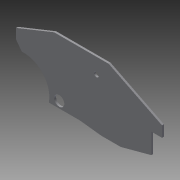
# Autodesk Inventor part: ShooterMountLeft_NERDS
Saved by Autodesk Inventor 2014 (Build 180170000, 170)
## iProperties
Created: 2016-01-30
Part Number: ShooterMountLeft_NERDS
Material: Generic
Document SubType Name: Modeling
Designer: bermudezr
Density: 1 g/cm^3
Appearance: Default
Author: bermudezr
Autodesk Inventor part; units mm, degrees
ref_plane "YZ Plane" through (0, 0, 0) normal (1, 0, 0) x (0, 1, 0)
ref_plane "XZ Plane" through (0, 0, 0) normal (0, 1, 0) x (-1, 0, 0)
ref_plane "XY Plane" through (0, 0, 0) normal (0, 0, 1) x (1, 0, 0)
sketch "Sketch1" plane through (0, 0, 0) normal (0, 0, 1) x (1, 0, 0)
  line L0 (-84.0821, 192.7052) -> (642.9929, 192.7052)
  line L1 (642.9929, 192.7052) -> (642.9929, -137.4948)
  line L2 (642.9929, -137.4948) -> (-84.0821, -137.4948)
  line L3 (-84.0821, -137.4948) -> (-84.0821, 192.7052)
  circle A0 centre (131.8179, -91.7748) radius 25.4
  circle A1 centre (318.0537, 116.5052) radius 12.7
  line L4 (642.9929, -137.4948) -> (592.1929, -137.4948)
  line L5 (592.1929, -137.4948) -> (592.1929, -73.9948)
  line L6 (592.1929, -73.9948) -> (642.9929, -73.9948)
  line L7 (642.9929, -73.9948) -> (642.9929, -137.4948)
  line L8 (642.9929, 192.7052) -> (592.6352, 192.7052)
  line L9 (642.9929, 2.2052) -> (642.9929, 192.7052)
  line L10 (-84.0821, 53.0052) -> (5.7204, 53.0052) construction
  line L11 (-84.0821, 65.7052) -> (68.3179, -137.4948)
  line L12 (595.3679, 192.7052) -> (595.3679, 2.2052)
  line L13 (595.3679, 2.2052) -> (642.9929, 2.2052)
  point P0 (0, 0)
  dimension "d0" = 727.075
  dimension "d2" = 50.8
  dimension "d3" = 25.4
  dimension "d4" = 215.9
  dimension "d5" = 279.4
  dimension "d14" = 152.4
  dimension "d15" = 203.2
  dimension "d16" = 330.2
  dimension "d17" = 63.5
  dimension "d19" = 50.8
  dimension "d20" = 139.7
  dimension "d21" = 45.72
  dimension "d22" = 254
  constraints: 28 end point, 5 parallel, 5 point on line, 4 horizontal, 3 perpendicular, 2 centre point
  measures "d0" distance of L1.end L2.end
  measures "d2" diameter of A0
  measures "d3" diameter of A1
  measures "d4" distance from line of L3 A0.centre
  measures "d5" distance of A1.centre A0.centre
  measures "d14" distance from line of L3 L11.end
  measures "d15" distance from line of L2 L11.start
  measures "d16" distance between parallel lines of L2 L0
  measures "d17" distance between parallel lines of L6 L2
  measures "d19" distance of L5.end L6.end
  measures "d20" distance between parallel lines of L13 L4
  measures "d21" distance from line of L2 A0.centre
  measures "d22" distance from line of L2 A1.centre
extrude "Extrusion1" add sketch "Sketch1" along normal blind 9.525 contours L0 L12 L13 L1 L6 L5 L2 L11 L3
sketch "Sketch3" plane through (0, 0, 9.525) normal (0, 0, 1) x (1, 0, 0)
  line L0 (595.3679, 2.2052) -> (595.3679, 192.7052) projected
  line L1 (595.3679, 192.7052) -> (-84.0821, 192.7052) projected
  line L2 (-84.0821, 192.7052) -> (-84.0821, 65.7052) projected
  line L3 (-84.0821, 116.5052) -> (106.4179, 192.7052)
  line L4 (595.3679, 2.2052) -> (684.2679, 2.2052)
  line L5 (684.2679, 2.2052) -> (684.2679, 40.3052)
  line L6 (684.2679, 40.3052) -> (595.3679, 40.3052)
  line L7 (595.3679, 40.3052) -> (595.3679, 2.2052)
  line L8 (684.2679, 40.3052) -> (379.4679, 192.7052)
  line L9 (595.3679, 40.3052) -> (595.3679, 84.7552)
  line L10 (595.3679, 84.7552) -> (595.3679, 192.7052)
  point P0 (0, 0)
  dimension "d32" = 190.5
  dimension "d33" = 76.2
  dimension "d38" = 88.9
  dimension "d39" = 38.1
  dimension "d40" = 215.9
  constraints: 16 end point, 5 point on line, 2 parallel, 1 collinear, 1 horizontal, 1 perpendicular
  measures "d32" distance from line of L2 L3.end
  measures "d33" distance from line of L1 L3.start
  measures "d38" distance of L6.end L5.end
  measures "d39" distance of L5.end L4.end
  measures "d40" distance of L0.end L8.end
extrude "Extrusion4" cut sketch "Sketch3" against normal blind 9.525 contours L8 L1 L0 | L0 L8 L6 | L3 L2 L1
sketch "Sketch4" plane through (0, 0, 9.525) normal (0, 0, 1) x (1, 0, 0)
  line L0 (595.3679, 2.2052) -> (595.3679, 84.7552) projected
  line L1 (595.3679, 84.7552) -> (379.4679, 192.7052) projected
  line L2 (595.3679, 84.7552) -> (684.2679, 40.3052)
  line L3 (684.2679, 40.3052) -> (595.3679, 40.3052)
  point P0 (0, 0)
  dimension "d43" = 88.9
  constraints: 4 end point, 1 collinear, 1 perpendicular, 1 point on line
  measures "d43" distance from line of L2.end L0
extrude "Extrusion5" add sketch "Sketch4" against normal blind 9.525
sketch "Sketch5" plane through (0, 0, 9.525) normal (0, 0, 1) x (1, 0, 0)
  line L0 (642.9929, 2.2052) -> (592.1929, 2.2052)
  line L1 (592.1929, 2.2052) -> (592.1929, -73.9948)
  line L2 (592.1929, -73.9948) -> (642.9929, -73.9948)
  line L3 (642.9929, -73.9948) -> (642.9929, 2.2052)
  point P0 (0, 0)
  constraints: 8 end point, 2 parallel, 1 horizontal, 1 perpendicular
extrude "Extrusion6" cut sketch "Sketch5" against normal blind 9.525
sketch "Sketch6" plane through (0, 0, 9.525) normal (0, 0, 1) x (1, 0, 0)
  line L0 (592.1929, -137.4948) -> (592.1929, 2.2052) projected
  line L1 (646.1679, 91.1052) -> (723.1394, 91.1052)
  line L2 (723.1394, 91.1052) -> (723.1394, -6.7385)
  line L3 (723.1394, -6.7385) -> (646.1679, -6.7385)
  line L4 (646.1679, -6.7385) -> (646.1679, 91.1052)
  line L5 (595.3679, 2.2052) -> (592.1929, 2.2052)
  line L6 (592.1929, 2.2052) -> (592.1929, 40.3052)
  line L7 (592.1929, 40.3052) -> (595.3679, 40.3052)
  line L8 (595.3679, 40.3052) -> (595.3679, 2.2052)
  point P0 (0, 0)
  dimension "d48" = 53.975
  constraints: 16 end point, 4 parallel, 2 horizontal, 2 perpendicular
  measures "d48" distance between parallel lines of L0 L4
extrude "Extrusion7" cut sketch "Sketch6" against normal blind 9.525
sketch "Sketch8" plane through (0, 0, 9.525) normal (0, 0, 1) x (1, 0, 0)
  line L0 (-84.0821, 65.7052) -> (68.3179, -137.4948) projected
  line L1 (68.3179, -137.4948) -> (592.1929, -137.4948) projected
  line L2 (592.1929, -137.4948) -> (592.1929, 40.3052) projected
  line L3 (592.1929, -96.6594) -> (439.7929, -137.4948)
  line L4 (341.7489, -137.4948) -> (170.3104, -117.1748)
  line L5 (170.3104, -117.1748) -> (53.0779, -117.1748)
  point P0 (0, 0)
  dimension "d51" = 152.4
  dimension "d52" = 165
  dimension "d53" = 98.044
  dimension "d54" = 20.32
  dimension "d60" = 173.24
  constraints: 6 end point, 4 point on line
  measures "d51" distance from line of L3.end L2
  measures "d52" angle of L1 L3
  measures "d53" distance of L3.end L4.start
  measures "d54" distance between parallel lines of L1 L5
  measures "d60" angle of L1 L4
extrude "Extrusion8" cut sketch "Sketch8" against normal blind 9.525
sketch "Sketch9" plane through (0, 0, 9.525) normal (0, 0, 1) x (1, 0, 0)
  line L0 (592.1929, -96.6594) -> (592.1929, 40.3052) projected
  line L1 (646.1679, 40.3052) -> (592.1929, 40.3052)
  line L2 (592.1929, 40.3052) -> (592.1929, 5.3802)
  line L3 (592.1929, 5.3802) -> (646.1679, 5.3802)
  line L4 (646.1679, 5.3802) -> (646.1679, 40.3052)
  point P0 (0, 0)
  dimension "d57" = 34.925
  constraints: 8 end point, 2 parallel, 1 horizontal, 1 perpendicular, 1 point on line
  measures "d57" distance of L2.end L1.end
extrude "Extrusion9" add sketch "Sketch9" against normal blind 9.525
sketch "Sketch10" plane through (0, 0, 9.525) normal (0, 0, 1) x (1, 0, 0)
  line L0 (-84.0821, 65.7052) -> (53.0779, -117.1748) projected
  line L1 (-84.0821, 116.5052) -> (-84.0821, 65.7052) projected
  line L2 (53.0779, -117.1748) -> (170.3104, -117.1748) projected
  arc A0 (81.0179, -117.1748) -> (-55.5071, 27.6052) centre (-44.6649, -98.9312) ccw
  point P0 (0, 0)
  point P1 (131.8179, -117.1748)
  dimension "d62" = 38.1
  dimension "d65" = 127
  dimension "d66" = 165.1
  constraints: 2 point on circle, 2 point on line, 1 centre point
  measures "d62" vertical distance of L0.start A0.end
  measures "d65" radius of A0
  measures "d66" distance from line of A0.start L1
extrude "Extrusion10" cut sketch "Sketch10" against normal blind 25.4
sketch "Sketch11" plane through (0, 0, 9.525) normal (0, 0, 1) x (1, 0, 0)
  arc A0 (81.0179, -117.1748) -> (-55.5071, 27.6052) centre (-44.6649, -98.9312) ccw projected
  line L0 (81.0179, -117.1748) -> (131.8179, -117.1748) projected
  line L1 (131.8179, -117.1748) -> (170.3104, -117.1748) projected
  line L2 (170.3104, -117.1748) -> (341.7489, -137.4948) projected
  line L3 (341.7489, -137.4948) -> (439.7929, -137.4948) projected
  line L4 (-84.0821, 116.5052) -> (-84.0821, 65.7052) projected
  line L5 (234.5998, -124.7948) -> (76.0086, -124.7948)
  line L6 (81.0179, -117.1748) -> (79.9118, -124.7948)
  point P0 (0, 0)
  point P1 (81.0179, -124.7948)
  dimension "d67" = 12.7
  constraints: 4 end point, 3 point on line, 1 perpendicular, 1 tangent
  measures "d67" distance between parallel lines of L3 L5
extrude "Extrusion11" add sketch "Sketch11" against normal blind 9.525
body "Solid1"
